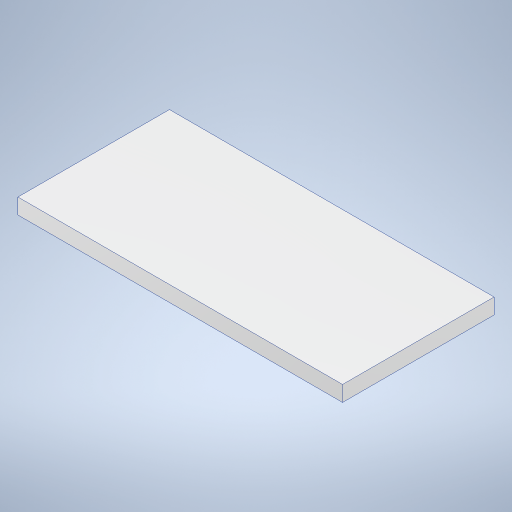
# Autodesk Inventor part: ZadBabkaOsnova
Saved by Autodesk Inventor 2024 (Build 280153000, 153)
## iProperties
Created: 2023-08-28
Part Number: ZadBabkaOsnova
Material: Aluminum 6061
Document SubType Name: Modeling
Designer: KirikDK
Density: 2.7 g/cm^3
Appearance: Aluminum - Flat
Mass: 3033.45 g
Surface Area: 1818.9 cm^2
Volume: 1123.5 cm^3
Author: KirikDK
Autodesk Inventor part; units mm, degrees
ref_plane "YZ Plane" through (0, 0, 0) normal (1, 0, 0) x (0, 1, 0)
ref_plane "XZ Plane" through (0, 0, 0) normal (0, 1, 0) x (-1, 0, 0)
ref_plane "XY Plane" through (0, 0, 0) normal (0, 0, 1) x (1, 0, 0)
sketch "Sketch1" plane through (0, 0, 0) normal (0, 1, 0) x (-1, 0, 0)
  line L0 (50, 50) -> (-125, 50)
  line L1 (-125, 50) -> (-125, -125)
  line L2 (-125, -125) -> (50, -125)
  line L3 (50, -125) -> (50, 50)
  point P0 (0, 0)
  dimension "d0" = 175
  dimension "d1" = 175
  constraints: 8 end point, 2 parallel, 1 horizontal, 1 perpendicular
  measures "d0" distance of L2.end L0.start
  measures "d1" distance of L0.start L0.end
extrude "Extrusion1" add sketch "Sketch1" along normal blind 12
sketch "Sketch2" plane through (0, 12, 0) normal (0, 1, 0) x (1, 0, 0)
  line L0 (-50, -50) -> (125, -50) projected
  line L1 (-150, -50) -> (225, -50)
  line L2 (225, -50) -> (225, 125)
  line L3 (225, 125) -> (-150, 125)
  line L4 (-150, 125) -> (-150, -50)
  line L5 (-50, 125) -> (-50, -50) projected
  line L6 (125, -50) -> (125, 125) projected
  point P0 (0, 0)
  point P1 (55, -50)
  dimension "d8" = 100
  dimension "d9" = 100
  constraints: 8 end point, 2 parallel, 1 horizontal, 1 perpendicular, 1 point on line
  measures "d8" distance between parallel lines of L6 L2
  measures "d9" distance between parallel lines of L5 L4
extrude "Extrusion2" add sketch "Sketch2" against normal blind 18
body "Solid1"
